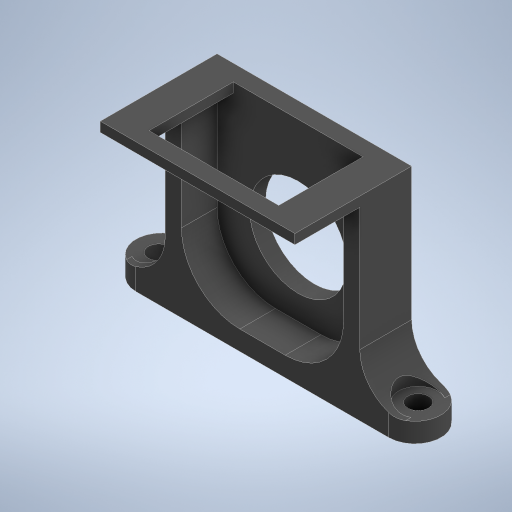
# Autodesk Inventor part: スイッチセッター
Saved by Autodesk Inventor 2024.1 (Build 281209000, 209)
## iProperties
Created: 2024-11-06
Part Number: スイッチセッター
Material: 一般
Document SubType Name: Modeling
Designer: hibik
Density: 1 g/cm^3
Appearance: 既定
Author: hibik
Autodesk Inventor part; units mm, degrees
ref_plane "YZ Plane" through (0, 0, 0) normal (1, 0, 0) x (0, 1, 0)
ref_plane "XZ Plane" through (0, 0, 0) normal (0, 1, 0) x (-1, 0, 0)
ref_plane "XY Plane" through (0, 0, 0) normal (0, 0, 1) x (1, 0, 0)
sketch "スケッチ1" plane through (0, 0, 0) normal (0, 0, 1) x (1, 0, 0)
  line L0 (-59, 0) -> (-38, 0)
  line L1 (-38, 0) -> (-38, -21)
  line L2 (-38, -21) -> (-59, -21)
  line L3 (-59, -21) -> (-59, 0)
  line L4 (-61, 2) -> (-36, 2)
  line L5 (-36, 2) -> (-36, -23)
  line L6 (-36, -23) -> (-61, -23)
  line L7 (-61, -23) -> (-61, 2)
  line L8 (-61, -23) -> (0, -23)
  line L9 (0, -23) -> (0, -17)
  line L10 (0, -17) -> (-61, -17)
  line L11 (-61, -17) -> (-61, -23)
  line L12 (-48.5, -23) -> (-85.5, -23)
  line L13 (-85.5, -23) -> (-85.5, -17)
  line L14 (-85.5, -17) -> (-48.5, -17)
  line L15 (-48.5, -17) -> (-48.5, -23)
  line L16 (-85.5, 1) -> (-82.5, 1)
  line L17 (-82.5, 1) -> (-82.5, -23)
  line L18 (-82.5, -23) -> (-85.5, -23)
  line L19 (-85.5, -23) -> (-85.5, 1)
  line L20 (-85.5, -17) -> (-90.7, -17)
  line L21 (-90.7, -17) -> (-90.7, -23)
  line L22 (-90.7, -23) -> (-85.5, -23)
  line L23 (-85.5, -23) -> (-85.5, -17)
  line L24 (-90.7, -23) -> (-93.7, -23)
  line L25 (-93.7, -23) -> (-93.7, 1)
  line L26 (-93.7, 1) -> (-90.7, 1)
  line L27 (-90.7, 1) -> (-90.7, -23)
  point P0 (0, 0)
  point P1 (-61, -10.5)
  point P2 (-59, -10.5)
  point P3 (-48.5, 2)
  point P4 (-48.5, 0)
  point P5 (-36, -17)
  point P6 (-82.5, -17)
  dimension "d0" = 21
  dimension "d1" = 21
  dimension "d4" = 38
  dimension "d5" = 25
  dimension "d6" = 6
  dimension "d31" = 37
  dimension "d33" = 5.2
  dimension "d34" = 3
  dimension "d35" = 18
  constraints: 56 end point, 14 parallel, 7 horizontal, 7 perpendicular, 6 point on line, 5 collinear, 4 midpoint, 2 equal length, 1 horizontal alignment, 1 vertical alignment
  measures "d0" distance of L1.end L2.end
  measures "d1" distance of L0.end L1.end
  measures "d4" distance from line of point (0, 0) L1
  measures "d5" distance of L4.start L4.end
  measures "d6" distance of L8.end L9.end
  measures "d31" distance of L12.start L12.end
  measures "d33" distance between parallel lines of L19 L27
  measures "d34" distance of L16.start L16.end
  measures "d35" distance between parallel lines of L14 L16
extrude "押し出し1" add sketch "スケッチ1" along normal blind 8 contours L10 L9 L8 L5
mirror "ミラー2" about plane through (0, -23, 0) normal (1, 0, 0)
sketch "スケッチ17" plane through (0, 0, 0) normal (0, 0, -1) x (-1, 0, 0)
  line L0 (-15, 13) -> (15, 13)
  line L1 (15, 13) -> (15, -17)
  line L2 (15, -17) -> (-15, -17)
  line L3 (-15, -17) -> (-15, 13)
  line L4 (-36, -17) -> (36, -17) projected
  point P0 (0, 13)
  point P1 (0, 13)
  point P2 (0, -17)
  dimension "d74" = 30
  dimension "d105" = 30
  constraints: 8 end point, 2 midpoint, 2 parallel, 1 coincident, 1 collinear, 1 horizontal, 1 perpendicular, 1 vertical alignment
  measures "d74" distance of L1.end L2.end
  measures "d105" distance of L0.end L1.end
extrude "押し出し16" add sketch "スケッチ17" against normal blind 18
sketch "スケッチ18" plane through (-15, 13, 0) normal (0, 1, 0) x (1, 0, 0)
  line L0 (5, -15.5) -> (25, -15.5)
  line L1 (25, -15.5) -> (25, -2.5)
  line L2 (25, -2.5) -> (5, -2.5)
  line L3 (5, -2.5) -> (5, -15.5)
  line L4 (0, 0) -> (30, 0) projected
  line L5 (0, 0) -> (0, -18) projected
  point P0 (15, 0)
  point P1 (15, -2.5)
  point P2 (15, 0)
  point P3 (5, -9)
  point P4 (0, -9)
  dimension "d77" = 20
  dimension "d78" = 13
  constraints: 8 end point, 4 midpoint, 2 parallel, 1 horizontal, 1 horizontal alignment, 1 perpendicular, 1 vertical alignment
  measures "d77" distance of L2.end L1.end
  measures "d78" distance of L1.end L0.end
extrude "押し出し17" cut sketch "スケッチ18" against normal up to surface (30 mm away)
sketch "スケッチ19" plane through (0, 0, 18) normal (0, 0, 1) x (1, 0, 0)
  line L0 (-15, -17) -> (-15, -23) projected
  line L1 (15, 13) -> (15, -17) projected
  line L2 (-15, -17) -> (15, -17)
  line L3 (15, -17) -> (15, 11.5)
  line L4 (15, 11.5) -> (-15, 11.5)
  line L5 (-15, 11.5) -> (-15, -17)
  line L6 (15, 13) -> (-15, 13) projected
  point P0 (0, 0)
  point P1 (-15, 13)
  point P2 (15, -17)
  dimension "d81" = 1.5
  constraints: 8 end point, 2 parallel, 1 horizontal, 1 perpendicular, 1 point on line, 1 other
extrude "押し出し18" cut sketch "スケッチ19" against normal up to surface (10 mm away)
sketch "スケッチ20" plane through (-15, 11.5, 8) normal (0, 0, 1) x (1, 0, 0)
  line L0 (0, 0) -> (30, 0) projected
  line L1 (30, -28.5) -> (51, -28.5) projected
  line L2 (2.5, 0) -> (47.5, 0)
  line L3 (40.5, -28.5) -> (2.5, -28.5)
  line L4 (2.5, -28.5) -> (2.5, 0)
  line L5 (5, 0) -> (5, -28.5) projected
  line L6 (25, 0) -> (27.5, 0)
  line L7 (27.5, 0) -> (27.5, -28.5)
  line L8 (27.5, -28.5) -> (25, -28.5)
  line L9 (25, -28.5) -> (25, 0)
  line L10 (25, -28.5) -> (25, 0) projected
  point P0 (15, -11.5)
  point P1 (40.5, -28.5)
  point P2 (25, -15)
  point P3 (5, -15)
  point P4 (51, -28.5)
  point P5 (5, -16)
  point P6 (25, -28.5)
  point P7 (27.5, 0)
  dimension "d85" = 2.5
  dimension "d113" = 2.5
  constraints: 12 end point, 3 horizontal, 2 parallel, 1 collinear, 1 midpoint, 1 perpendicular, 1 point on line, 6 other
  measures "d85" distance between parallel lines of L4 L5
  measures "d113" distance between parallel lines of L7 L9
extrude "押し出し19" cut sketch "スケッチ20" against normal up to surface (5.5 mm away) contours L0 L5 L3 L4 | L0 L7 L3 L9
sketch "スケッチ21" plane through (-10, 13, 2.5) normal (0, 0, 1) x (1, 0, 0)
  line L0 (20, 0) -> (20, -1.5) projected
  line L1 (0, 0) -> (20, 0) projected
  line L2 (0, 0) -> (0, -1.5) projected
  line L3 (-2.5, -30) -> (22.5, -30) projected
  circle A0 centre (10, -15.75) radius 7.5
  line L4 (-5, -1.5) -> (25, -1.5) projected
  line L5 (-2.5, -30) -> (-2.5, -1.5) projected
  line L6 (22.5, -30) -> (22.5, -1.5) projected
  line L7 (22.5, -1.5) -> (20, -1.5) projected
  line L8 (0, -1.5) -> (-2.5, -1.5) projected
  line L9 (-2.5, -1.5) -> (-2.5, -30) projected
  point P0 (0, -2)
  point P1 (10, -1.5)
  point P2 (25, -1.5)
  point P3 (-2.5, -15.75)
  dimension "d89" = 15
  constraints: 1 centre point, 1 horizontal alignment, 1 midpoint, 1 vertical alignment, 2 other
  measures "d89" diameter of A0
extrude "押し出し20" cut sketch "スケッチ21" against normal through all contours A0
sketch "スケッチ26" plane through (-36, -23, 0) normal (0, -1, 0) x (1, 0, 0)
  line L0 (0, 0) -> (72, 0) projected
  line L1 (72, 0) -> (72, 8) projected
  line L2 (0, 8) -> (72, 8) projected
  line L3 (0, 0) -> (0, 8) projected
  point P0 (36, 0)
extrude "押し出し25" cut sketch "スケッチ26" against normal up to surface (6 mm away)
sketch "スケッチ27" plane through (-15, -17, 0) normal (0, -1, 0) x (1, 0, 0)
  line L0 (-8.5, 8) -> (38.5, 8)
  line L1 (38.5, 8) -> (38.5, 0)
  line L2 (38.5, 0) -> (-8.5, 0)
  line L3 (-8.5, 0) -> (-8.5, 8)
  line L4 (-5, 8) -> (35, 8)
  line L5 (35, 8) -> (35, 0) construction
  line L6 (35, 0) -> (-5, 0)
  line L7 (-5, 0) -> (-5, 8) construction
  line L8 (0, 8) -> (30, 8) projected
  line L9 (30, 0) -> (0, 0) projected
  circle A0 centre (-5, 4) radius 1.6
  circle A1 centre (35, 4) radius 1.6
  point P0 (15, 0)
  point P1 (10.6, 8)
  point P2 (15, 0)
  point P3 (15, 0)
  dimension "d108" = 40
  dimension "d109" = 47
  dimension "d110" = 3.2
  constraints: 16 end point, 6 midpoint, 4 parallel, 2 centre point, 2 collinear, 2 horizontal, 2 perpendicular, 1 equal radius, 1 point on line
  measures "d108" distance between parallel lines of L5 L7
  measures "d109" distance of L0.start L0.end
  measures "d110" diameter of A0
extrude "押し出し26" add sketch "スケッチ27" against normal blind 3
fillet "フィレット6" radius 6.5 2 edges at (-15, -14, 4) (15, -14, 4)
sketch "スケッチ28" plane through (-15, -14, 0) normal (0, 1, 0) x (1, 0, 0)
  circle A0 centre (-5, -4) radius 1.6 projected
  circle A1 centre (35, -4) radius 1.6 projected
  line L0 (-8.5, -8) -> (38.5, -8) projected
  line L1 (-8.5, -8) -> (-8.5, 0) projected
  line L2 (38.5, 0) -> (-8.5, 0) projected
  line L3 (38.5, 0) -> (38.5, -8) projected
  circle A2 centre (35, -4) radius 3
  circle A3 centre (-5, -4) radius 3
  point P0 (15, 0)
  dimension "d116" = 6
  constraints: 2 centre point, 2 coincident, 1 equal radius
  measures "d116" diameter of A2
extrude "押し出し27" cut sketch "スケッチ28" along normal through all contours A0 | A1 | A2 | A3
fillet "フィレット7" radius 4 4 edges at (-23.5, -15.5, 8) (-23.5, -15.5, 0) (23.5, -15.5, 8) (23.5, -15.5, 0)
fillet "フィレット8" radius 9 2 edges at (12.5, -14, 5.25) (-12.5, -14, 5.25)
equation "\"d0\" = d1"
equation "\"d113\" = d85"
